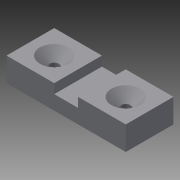
# Autodesk Inventor part: CameraArmMount
Saved by Autodesk Inventor 2015 (Build 190159000, 159)
## iProperties
Created: 2015-11-25
Part Number: CameraArmMount
Material: Generic
Document SubType Name: Modeling
Designer: Lauszus
Density: 1 g/cm^3
Appearance: Default
Author: Lauszus
Autodesk Inventor part; units mm, degrees
ref_plane "YZ Plane" through (0, 0, 0) normal (1, 0, 0) x (0, 1, 0)
ref_plane "XZ Plane" through (0, 0, 0) normal (0, 1, 0) x (-1, 0, 0)
ref_plane "XY Plane" through (0, 0, 0) normal (0, 0, 1) x (1, 0, 0)
sketch "Sketch1" plane through (0, 0, 0) normal (0, 0, 1) x (1, 0, 0)
  line L0 (-15.1742, 2.0557) -> (9.8258, 2.0557)
  line L1 (9.8258, 2.0557) -> (9.8258, -7.9443)
  line L2 (9.8258, -7.9443) -> (-15.1742, -7.9443)
  line L3 (-15.1742, -7.9443) -> (-15.1742, 2.0557)
  point P0 (0, 0)
  dimension "d0" = 25
  dimension "d1" = 10
  constraints: 8 end point, 2 parallel, 1 horizontal, 1 perpendicular
  measures "d0" distance of L0.start L0.end
  measures "d1" distance of L0.end L1.end
extrude "Extrusion1" add sketch "Sketch1" along normal blind 5
sketch "Sketch2" plane through (0, 0, 5) normal (0, 0, 1) x (1, 0, 0)
  circle A0 centre (-10.1742, -2.9443) radius 1
  line L0 (-15.1742, 2.0557) -> (-15.1742, -7.9443) projected
  line L1 (9.8258, 2.0557) -> (-15.1742, 2.0557) projected
  line L2 (-2.6742, 2.0557) -> (-2.6742, -2.9443)
  circle A1 centre (4.8258, -2.9443) radius 1
  point P0 (0, 0)
  dimension "d4" = 2
  dimension "d5" = 5
  dimension "d6" = 5
  constraints: 2 centre point, 2 end point, 1 midpoint, 1 symmetric about line, 1 vertical, 1 other
  measures "d4" diameter of A0
  measures "d5" distance from line of L0 A0.centre
  measures "d6" distance from line of A0.centre L1
hole "Hole1" at (-10.1742, -2.9443, 5) at (4.8258, -2.9443, 5) direction (0, 0, -1) diameter 2 end through all countersink diameter 6 countersink angle 90
sketch "Sketch3" plane through (0, 0, 5) normal (0, 0, 1) x (1, 0, 0)
  line L0 (9.8258, 2.0557) -> (-15.1742, 2.0557) projected
  line L1 (-15.1742, -7.9443) -> (9.8258, -7.9443) projected
  line L2 (-5.1742, 2.0557) -> (-0.1742, 2.0557)
  line L3 (-0.1742, 2.0557) -> (-0.1742, -7.9443)
  line L4 (-0.1742, -7.9443) -> (-5.1742, -7.9443)
  line L5 (-5.1742, -7.9443) -> (-5.1742, 2.0557)
  line L6 (-15.1742, 2.0557) -> (-15.1742, -7.9443) projected
  line L7 (9.8258, -7.9443) -> (9.8258, 2.0557) projected
  point P0 (0, 0)
  dimension "d14" = 10
  dimension "d15" = 10
  constraints: 8 end point, 2 parallel, 2 point on line, 1 horizontal, 1 perpendicular
  measures "d14" distance between parallel lines of L6 L5
  measures "d15" distance between parallel lines of L7 L3
extrude "Extrusion2" cut sketch "Sketch3" against normal blind 2 contours L3 L1 L5 L0
body "Solid1"
